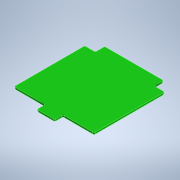
# Autodesk Inventor part: MainBoard
Saved by Autodesk Inventor 2021 (Build 250183000, 183)
## iProperties
Created: 2021-05-13
Part Number: MainBoard
Material: Generic
Document SubType Name: Modeling
Designer: ermoz
Density: 1 g/cm^3
Appearance: Default
Author: ermoz
Autodesk Inventor part; units mm, degrees
ref_plane "YZ Plane" through (0, 0, 0) normal (1, 0, 0) x (0, 1, 0)
ref_plane "XZ Plane" through (0, 0, 0) normal (0, 1, 0) x (-1, 0, 0)
ref_plane "XY Plane" through (0, 0, 0) normal (0, 0, 1) x (1, 0, 0)
sketch "Sketch1" plane through (0, 0, 0) normal (0, 1, 0) x (-1, 0, 0)
  line L0 (-25, -37.5) -> (25, -37.5)
  line L1 (25, -37.5) -> (25, 30.5)
  line L2 (25, 30.5) -> (-25, 30.5)
  line L3 (-25, 30.5) -> (-25, -37.5)
  line L4 (-25, -37.5) -> (25, 30.5) construction
  line L5 (25, -37.5) -> (-25, 30.5) construction
  point P0 (0, -3.5)
  point P1 (0, -3.5)
  point P2 (0, -3.5)
  dimension "d2" = 1.6
  dimension "d0" = 68
  dimension "d1" = 50
  constraints: 12 end point, 4 midpoint, 2 horizontal, 2 parallel, 1 perpendicular
  measures "d0" distance of L0.end L1.end
  measures "d1" distance of L1.end L2.end
extrude "Extrusion1" add sketch "Sketch1" along normal blind 1.6
sketch "Sketch2" plane through (0, 0, 0) normal (0, -1, 0) x (1, 0, 0)
  line L0 (25, 30.5) -> (25, -37.5) projected
  line L1 (25, -29.5) -> (34, -29.5)
  line L2 (34, -29.5) -> (34, 30.5)
  line L3 (34, 30.5) -> (25, 30.5)
  line L4 (25, 30.5) -> (25, -29.5)
  line L5 (-25, -37.5) -> (-25, 30.5) projected
  line L6 (-25, -29.5) -> (-34, -29.5)
  line L7 (-34, -29.5) -> (-34, 30.5)
  line L8 (-34, 30.5) -> (-25, 30.5)
  line L9 (-25, 30.5) -> (-25, -29.5)
  line L10 (25, -37.5) -> (-25, -37.5) projected
  line L11 (-7.5, 37.5) -> (7.5, 37.5)
  line L12 (7.5, 37.5) -> (7.5, 30.5)
  line L13 (7.5, 30.5) -> (-7.5, 30.5)
  line L14 (-7.5, 30.5) -> (-7.5, 37.5)
  line L15 (-7.5, 37.5) -> (7.5, 30.5) construction
  line L16 (7.5, 37.5) -> (-7.5, 30.5) construction
  line L17 (-25, 30.5) -> (25, 30.5) projected
  point P0 (0, 0)
  point P1 (25, 28.5)
  point P2 (25, -35.5)
  point P3 (-25, -35.5)
  point P4 (-25, 28.5)
  point P5 (-23, 30.5)
  point P6 (23, 30.5)
  point P7 (23, -37.5)
  point P8 (-23, -37.5)
  point P9 (25, 23.5)
  point P10 (-25, 23.5)
  point P11 (25, 28.5)
  point P12 (-25, 28.5)
  point P13 (0, 34)
  point P14 (0, 34)
  point P15 (0, 30.5)
  dimension "d5" = 9
  dimension "d6" = 9
  dimension "d8" = 8
  dimension "d12" = 15
  dimension "d13" = 7
  constraints: 28 end point, 6 parallel, 4 midpoint, 4 point on line, 3 horizontal, 3 perpendicular, 1 collinear, 1 vertical alignment
  measures "d5" distance of L0.start L2.end
  measures "d6" distance of L7.end L5.end
  measures "d8" distance between parallel lines of L10 L6
  measures "d12" distance of L12.end L13.end
  measures "d13" distance of L11.end L12.end
extrude "Extrusion2" add sketch "Sketch2" against normal up to surface (1.6 mm away) contours L3 L2 L1 L0 | L13 L14 L11 L12 | L5 L6 L7 L8
fillet "Fillet2" radius 1 12 edges at (-34, 0.8, 30.5) (-25, 0.8, -29.5) (-34, 0.8, -29.5) (25, 0.8, -29.5) (34, 0.8, -29.5) (34, 0.8, 30.5) (25, 0.8, -37.5) (-25, 0.8, -37.5) (7.5, 0.8, 30.5) (7.5, 0.8, 37.5) (-7.5, 0.8, 37.5) (-7.5, 0.8, 30.5)
body "Solid1"
